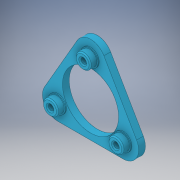
# Autodesk Inventor part: Bottom
Saved by Autodesk Inventor 2019.1 (Build 231200000, 200)
## iProperties
Created: 2019-01-01
Part Number: Bottom
Material: Generisch
Document SubType Name: Modeling
Designer: JochenAlt
Density: 1 g/cm^3
Appearance: Vorgabe
Author: JochenAlt
Autodesk Inventor part; units mm, degrees
ref_plane "YZ Plane" through (0, 0, 0) normal (1, 0, 0) x (0, 1, 0)
ref_plane "XZ Plane" through (0, 0, 0) normal (0, 1, 0) x (-1, 0, 0)
ref_plane "XY Plane" through (0, 0, 0) normal (0, 0, 1) x (1, 0, 0)
sketch "Skizze1" plane through (0, 0, 0) normal (0, 0, 1) x (1, 0, 0)
  circle A0 centre (0, 0) radius 16.8 construction
  line L0 (0, 31.7725) -> (0, -25.085) construction
  circle A1 centre (0, 16.8) radius 1.25
  circle A2 centre (14.5492, -8.4) radius 1.25
  circle A3 centre (-14.5492, -8.4) radius 1.25
  line L1 (0, 16.8) -> (14.5492, -8.4) construction
  line L2 (-14.5492, -8.4) -> (14.5492, -8.4) construction
  line L3 (-14.5492, -8.4) -> (0, 16.8) construction
  line L4 (5.9323, 20.225) -> (20.4815, -4.975)
  line L5 (14.5492, -15.25) -> (-14.5492, -15.25)
  line L6 (-20.4815, -4.975) -> (-5.9323, 20.225)
  arc A4 (-20.4815, -4.975) -> (-14.5492, -15.25) centre (-14.5492, -8.4) ccw
  arc A5 (14.5492, -15.25) -> (20.4815, -4.975) centre (14.5492, -8.4) ccw
  arc A6 (5.9323, 20.225) -> (-5.9323, 20.225) centre (0, 16.8) ccw
  circle A7 centre (0, 16.8) radius 3.35
  circle A8 centre (-14.5492, -8.4) radius 3.35
  circle A9 centre (14.5492, -8.4) radius 3.35
  circle A10 centre (0, 16.8) radius 3.85
  circle A11 centre (14.5492, -8.4) radius 3.85
  circle A12 centre (-14.5492, -8.4) radius 3.85
  circle A13 centre (0, 0) radius 12.5
  circle A14 centre (0, 16.8) radius 2.5
  circle A15 centre (-14.5492, -8.4) radius 2.5
  circle A16 centre (14.5492, -8.4) radius 2.5
  point P0 (0, 12.95)
  point P1 (0, 12.5)
  dimension "d19" = 12.5
  dimension "d1" = 2.5
  dimension "d2" = 16.8
  dimension "d3" = 0.5
  dimension "d4" = 6.7
  dimension "d5" = 3
  dimension "d16" = 5
  constraints: 15 centre point, 14 coincident, 12 end point, 9 equal radius, 9 point on circle, 6 tangent, 3 point on line, 2 equal length, 2 vertical alignment, 5 other
  measures "d1" diameter of A1
  measures "d2" radius of A0
  measures "d4" diameter of A7
  measures "d16" diameter of A14
extrude "Extrusion1" add sketch "Skizze1" along normal blind 3 contours L4 A5 L5 A4 L6 A6 | A7 | A8 | A9 | A10 | A11 | A12 | A14 | A15 | A16
extrude "Extrusion2" add sketch "Skizze1" along normal blind 0.5 from surface at 3 contours A7 | A8 | A9 | A10 | A11 | A12 | A14 | A15 | A16
extrude "Extrusion3" add sketch "Skizze1" along normal blind 3 from surface at 3.5 contours A7 | A8 | A9 | A14 | A15 | A16
chamfer "Fase1" distance 0.5 angle 45 6 edges at (-3.35, 16.8, 6.5) (-17.8992, -8.4, 6.5) (11.1992, -8.4, 6.5) (-1.25, 16.8, 6.5) (-15.7992, -8.4, 6.5) (13.2992, -8.4, 6.5)
extrude "Extrusion4" cut sketch "Skizze1" along normal blind 2 contours A14 | A15 | A16
